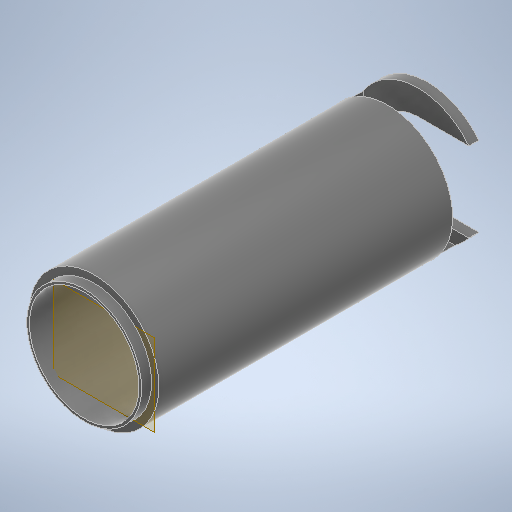
# Autodesk Inventor part: Magazine_Tube_2
Saved by Autodesk Inventor 2025.1 (Build 291241020, 241B)
## iProperties
Created: 2024-11-13
Part Number: Magazine_Tube_2
Material: PC/ABS Plastic
Document SubType Name: Modeling
Designer: leon-
Density: 1.1 g/cm^3
Appearance: Smooth - Black
Author: leon-
## iProperties of the stored document Magazine_Tube_2_3DPrint.ipt
Created: 2024-11-14
Part Number: Magazine_Tube_2_3DPrint
Material: Generic
Document SubType Name: Modeling
Designer: leon-
Density: 1 g/cm^3
Appearance: Default
Author: leon-
Autodesk Inventor part; units mm, degrees
ref_plane "YZ Plane" through (0, 0, 0) normal (1, 0, 0) x (0, 1, 0)
ref_plane "XZ Plane" through (0, 0, 0) normal (0, 1, 0) x (-1, 0, 0)
ref_plane "XY Plane" through (0, 0, 0) normal (0, 0, 1) x (1, 0, 0)
sketch "Sketch1" plane through (0, 0, 0) normal (0, 0, 1) x (1, 0, 0)
  circle A0 centre (0, 0) radius 16.5
  circle A1 centre (0, 0) radius 19.5
  dimension "d0" = 33
  dimension "d1" = 39
  constraints: 2 centre point, 2 coincident
  measures "d0" diameter of A0
  measures "d1" diameter of A1
extrude "Extrusion1" add sketch "Sketch1" along normal blind 195
ref_plane "Work Plane1" through (0, 0, 97.5) normal (0, 0, 1) x (1, 0, 0)
sketch "Sketch2" plane through (0, 0, 195) normal (0, 0, 1) x (1, 0, 0)
  circle A0 centre (0, 0) radius 19.5 projected
extrude "Extrusion2" add sketch "Sketch2" along normal blind 3
mirror "Mirror1" about plane through (0, 0, 97.5) normal (0, 0, 1) of "Extrusion2"
sketch "Sketch5" plane through (0, 0, -3) normal (0, 0, -1) x (-1, 0, 0)
  circle A0 centre (0, 0) radius 12
  dimension "d12" = 24
  constraints: 1 centre point, 1 coincident
  measures "d12" diameter of A0
extrude "Extrusion5" cut sketch "Sketch5" against normal blind 10
sketch "Sketch6" plane through (0, 0, 0) normal (1, 0, 0) x (0, 1, 0)
  line L0 (12, -3) -> (-12, -3) projected
  line L1 (-12, 0) -> (12, 0) projected
  line L2 (12, 0) -> (-12, 0)
  line L3 (-12, 0) -> (-12, -3)
  line L4 (-12, -3) -> (12, -3)
  line L5 (12, -3) -> (12, 0)
  point P0 (0, 0)
  constraints: 8 end point, 2 parallel, 1 horizontal, 1 perpendicular
extrude "Extrusion6" cut sketch "Sketch6" along normal through all
sketch "Sketch7" plane through (0, 0, 0) normal (1, 0, 0) x (0, 1, 0)
  line L0 (-16.5, 0) -> (16.5, 0) projected
  line L1 (16.5, 0) -> (-16, 0)
  line L2 (-16, 0) -> (-16, 9)
  line L3 (-16, 9) -> (16.5, 9)
  line L4 (16.5, 9) -> (16.5, 0)
  point P0 (0, 0)
  point P1 (-12, 0)
  point P2 (12, 0)
  dimension "d17" = 9
  constraints: 8 end point, 2 parallel, 1 horizontal, 1 perpendicular
  measures "d17" distance between parallel lines of L0 L3
extrude "Extrusion7" cut sketch "Sketch7" along normal through all
sketch "Sketch8" plane through (0, 0, 195) normal (0, 0, -1) x (-1, 0, 0)
  circle A0 centre (0, 0) radius 10
  circle A1 centre (0, 0) radius 19.5
  circle A2 centre (0, 0) radius 19.5 projected
  dimension "d20" = 20
  constraints: 2 centre point, 2 coincident, 1 concentric
  measures "d20" diameter of A0
extrude "Extrusion8" add sketch "Sketch8" along normal blind 5
sketch "Sketch9" plane through (0, 0, 97.5) normal (0, 0, 1) x (1, 0, 0)
  circle A0 centre (0, 0) radius 19.5 projected
extrude "Extrusion9" cut sketch "Sketch9" along normal through all
sketch "Sketch10" plane through (0, 0, 97.5) normal (0, 0, 1) x (1, 0, 0)
  circle A0 centre (0, 0) radius 16.5
  circle A1 centre (0, 0) radius 17.3
  dimension "d25" = 0.8
  dimension "d26" = 33
  constraints: 2 centre point, 2 coincident
  measures "d25" radial gap between concentric circles of A1 A0
  measures "d26" diameter of A0
extrude "Extrusion10" add sketch "Sketch10" along normal blind 3
sketch "Sketch12" plane through (0, 0, 0) normal (0, 1, 0) x (-1, 0, 0)
  line L0 (-16.5, 9) -> (0, 9) projected
  line L1 (-15.3704, 0) -> (0, 0) projected
  line L2 (16.5, 100.5) -> (16.5, 0) projected
  line L3 (16.5, 9) -> (-16.5, 9)
  line L4 (-16.5, 9) -> (-16.5, 0)
  line L5 (-16.5, 0) -> (16.5, 0)
  line L6 (16.5, 0) -> (16.5, 9)
  line L7 (-16.5, 100.5) -> (-16.5, 9) projected
  point P0 (-4.0311, 9)
  point P1 (-16.5, 9)
  constraints: 8 end point, 3 collinear, 2 parallel, 1 horizontal, 1 perpendicular, 1 point on line
extrude "Extrusion12" cut sketch "Sketch12" along normal through all
body "Solid1"
